Autodesk Inventor part; units mm, degrees
(part 7 of 8)
  spline S187 degree 3 poles (3.4162, -6.9877) (3.4167, -6.9758) (3.4179, -6.9524) (3.4233, -6.9183) (3.431, -6.8857) (3.4418, -6.8549) (3.4554, -6.8256) (3.4716, -6.7979) (3.4908, -6.7719) (3.5125, -6.7478) (3.5362, -6.7258) (3.5617, -6.7067) (3.5885, -6.6906) (3.6165, -6.6772) (3.6461, -6.6671) (3.6769, -6.6596) (3.7092, -6.6551) (3.7311, -6.6546) (3.7423, -6.6544) knots 0 0 0 0 0.068791 0.135103 0.198979 0.261904 0.323495 0.385195 0.446969 0.509765 0.572251 0.633405 0.693251 0.752583 0.812579 0.873275 0.93555 1 1 1 1
  spline S188 degree 3 poles (3.7423, -6.6544) (3.7532, -6.6546) (3.7748, -6.6551) (3.8062, -6.6595) (3.8362, -6.6662) (3.8645, -6.6758) (3.8911, -6.6886) (3.9161, -6.7039) (3.9398, -6.7217) (3.9611, -6.7426) (3.9807, -6.765) (3.9975, -6.7888) (4.012, -6.8135) (4.0241, -6.8391) (4.0329, -6.8659) (4.0397, -6.8935) (4.0435, -6.9223) (4.0441, -6.9417) (4.0444, -6.9516) knots 0 0 0 0 0.069475 0.136517 0.200789 0.26383 0.325735 0.387291 0.449509 0.512968 0.576275 0.63758 0.697903 0.757172 0.816599 0.876653 0.93729 1 1 1 1
  spline S189 degree 3 poles (4.0444, -6.9516) (4.0439, -6.9656) (4.0429, -6.9932) (4.0347, -7.0337) (4.0219, -7.0731) (4.0065, -7.1047) (3.9909, -7.1302) (3.9769, -7.1512) (3.9605, -7.1738) (3.9414, -7.1979) (3.9201, -7.2238) (3.8964, -7.2514) (3.8701, -7.2803) (3.8516, -7.3001) (3.842, -7.3104) knots 0 0 0 0 0.098702 0.195672 0.292422 0.391343 0.444462 0.504229 0.570352 0.642546 0.722288 0.807921 0.90047 1 1 1 1
  line L208 (3.842, -7.3104) -> (3.5918, -7.5774)
  line L209 (3.5918, -7.5774) -> (4.0572, -7.5774)
  line L210 (4.0572, -7.5774) -> (4.0572, -7.68)
  line L211 (4.0572, -7.68) -> (3.3777, -7.68)
  line L212 (3.3777, -7.68) -> (3.7655, -7.2661)
  spline S190 degree 3 poles (3.7655, -7.2661) (3.775, -7.2563) (3.7931, -7.2373) (3.8187, -7.2097) (3.8418, -7.1841) (3.8624, -7.1605) (3.88, -7.1386) (3.8957, -7.1191) (3.9083, -7.1012) (3.9219, -7.0804) (3.9351, -7.055) (3.9464, -7.024) (3.9534, -6.9921) (3.9542, -6.9705) (3.9546, -6.9596) knots 0 0 0 0 0.110803 0.212829 0.306101 0.390647 0.466924 0.534481 0.593587 0.644557 0.7362 0.825024 0.911986 1 1 1 1
  spline S191 degree 3 poles (3.1854, -6.9596) (3.1852, -6.9528) (3.1848, -6.9394) (3.1817, -6.9197) (3.1769, -6.9006) (3.1701, -6.8823) (3.161, -6.8647) (3.15, -6.848) (3.1374, -6.8318) (3.1227, -6.8166) (3.1066, -6.8027) (3.0895, -6.7903) (3.0715, -6.78) (3.0526, -6.7716) (3.0328, -6.765) (3.0121, -6.7604) (2.9906, -6.7575) (2.9759, -6.7571) (2.9684, -6.7569) knots 0 0 0 0 0.061965 0.122122 0.180988 0.239933 0.299906 0.359989 0.421776 0.486576 0.551535 0.615018 0.677259 0.73973 0.80305 0.866495 0.931973 1 1 1 1
  spline S192 degree 3 poles (2.9684, -6.7569) (2.9606, -6.7571) (2.9453, -6.7575) (2.9227, -6.7603) (2.9012, -6.7652) (2.8807, -6.7718) (2.8611, -6.7802) (2.8426, -6.7907) (2.8251, -6.8032) (2.8087, -6.8174) (2.7936, -6.8332) (2.7804, -6.8508) (2.7688, -6.8699) (2.7586, -6.8904) (2.7504, -6.9126) (2.7441, -6.9363) (2.7392, -6.9614) (2.7375, -6.9788) (2.7367, -6.9877) knots 0 0 0 0 0.064439 0.126547 0.186887 0.245878 0.304041 0.362191 0.420976 0.48066 0.5406 0.600689 0.661936 0.724443 0.789038 0.856314 0.926352 1 1 1 1
  line L213 (2.7367, -6.9877) -> (2.6469, -6.9877)
  spline S193 degree 3 poles (2.6469, -6.9877) (2.6475, -6.9758) (2.6487, -6.9524) (2.654, -6.9183) (2.6617, -6.8857) (2.6726, -6.8549) (2.6861, -6.8256) (2.7023, -6.7979) (2.7215, -6.7719) (2.7433, -6.7478) (2.767, -6.7258) (2.7925, -6.7067) (2.8193, -6.6906) (2.8473, -6.6772) (2.8769, -6.6671) (2.9077, -6.6596) (2.9399, -6.6551) (2.9619, -6.6546) (2.973, -6.6544) knots 0 0 0 0 0.068791 0.135103 0.198979 0.261904 0.323495 0.385195 0.446969 0.509765 0.572251 0.633405 0.693251 0.752583 0.812579 0.873275 0.93555 1 1 1 1
  spline S194 degree 3 poles (2.973, -6.6544) (2.984, -6.6546) (3.0056, -6.6551) (3.037, -6.6595) (3.0669, -6.6662) (3.0953, -6.6758) (3.1219, -6.6886) (3.1469, -6.7039) (3.1705, -6.7217) (3.1919, -6.7426) (3.2114, -6.765) (3.2283, -6.7888) (3.2428, -6.8135) (3.2548, -6.8391) (3.2637, -6.8659) (3.2704, -6.8935) (3.2742, -6.9223) (3.2748, -6.9417) (3.2751, -6.9516) knots 0 0 0 0 0.069475 0.136517 0.200789 0.26383 0.325735 0.387291 0.449509 0.512968 0.576275 0.63758 0.697903 0.757172 0.816599 0.876653 0.93729 1 1 1 1
  spline S195 degree 3 poles (3.2751, -6.9516) (3.2746, -6.9656) (3.2737, -6.9932) (3.2655, -7.0337) (3.2527, -7.0731) (3.2372, -7.1047) (3.2217, -7.1302) (3.2077, -7.1512) (3.1912, -7.1738) (3.1722, -7.1979) (3.1509, -7.2238) (3.1272, -7.2514) (3.1009, -7.2803) (3.0824, -7.3001) (3.0728, -7.3104) knots 0 0 0 0 0.098702 0.195672 0.292422 0.391343 0.444462 0.504229 0.570352 0.642546 0.722288 0.807921 0.90047 1 1 1 1
  line L214 (3.0728, -7.3104) -> (2.8226, -7.5774)
  line L215 (2.8226, -7.5774) -> (3.2879, -7.5774)
  line L216 (3.2879, -7.5774) -> (3.2879, -7.68)
  line L217 (3.2879, -7.68) -> (2.6085, -7.68)
  line L218 (2.6085, -7.68) -> (2.9963, -7.2661)
  spline S196 degree 3 poles (2.9963, -7.2661) (3.0057, -7.2563) (3.0239, -7.2373) (3.0495, -7.2097) (3.0726, -7.1841) (3.0931, -7.1605) (3.1108, -7.1386) (3.1265, -7.1191) (3.139, -7.1012) (3.1527, -7.0804) (3.1659, -7.055) (3.1772, -7.024) (3.1841, -6.9921) (3.185, -6.9705) (3.1854, -6.9596) knots 0 0 0 0 0.110803 0.212829 0.306101 0.390647 0.466924 0.534481 0.593587 0.644557 0.7362 0.825024 0.911986 1 1 1 1
  spline S197 degree 3 poles (7.9546, -4.4196) (7.9544, -4.4128) (7.9541, -4.3994) (7.9509, -4.3797) (7.9461, -4.3606) (7.9393, -4.3423) (7.9303, -4.3247) (7.9193, -4.308) (7.9066, -4.2918) (7.8919, -4.2766) (7.8758, -4.2627) (7.8588, -4.2503) (7.8408, -4.24) (7.8218, -4.2316) (7.8021, -4.225) (7.7814, -4.2204) (7.7599, -4.2175) (7.7452, -4.2171) (7.7377, -4.2169) knots 0 0 0 0 0.061965 0.122122 0.180988 0.239933 0.299906 0.359989 0.421776 0.486576 0.551535 0.615018 0.677259 0.73973 0.80305 0.866495 0.931973 1 1 1 1
  spline S198 degree 3 poles (7.7377, -4.2169) (7.7298, -4.2171) (7.7145, -4.2175) (7.6919, -4.2203) (7.6704, -4.2252) (7.6499, -4.2318) (7.6303, -4.2402) (7.6118, -4.2507) (7.5943, -4.2632) (7.578, -4.2774) (7.5629, -4.2932) (7.5496, -4.3108) (7.538, -4.3299) (7.5279, -4.3504) (7.5197, -4.3726) (7.5134, -4.3963) (7.5084, -4.4214) (7.5067, -4.4388) (7.5059, -4.4477) knots 0 0 0 0 0.064439 0.126547 0.186887 0.245878 0.304041 0.362191 0.420976 0.48066 0.5406 0.600689 0.661936 0.724443 0.789038 0.856314 0.926352 1 1 1 1
  line L219 (7.5059, -4.4477) -> (7.4162, -4.4477)
  spline S199 degree 3 poles (7.4162, -4.4477) (7.4167, -4.4358) (7.4179, -4.4124) (7.4233, -4.3783) (7.431, -4.3457) (7.4418, -4.3149) (7.4554, -4.2856) (7.4716, -4.2579) (7.4908, -4.2319) (7.5125, -4.2078) (7.5362, -4.1858) (7.5617, -4.1667) (7.5885, -4.1506) (7.6165, -4.1372) (7.6461, -4.1271) (7.6769, -4.1196) (7.7092, -4.1151) (7.7311, -4.1146) (7.7423, -4.1144) knots 0 0 0 0 0.068791 0.135103 0.198979 0.261904 0.323495 0.385195 0.446969 0.509765 0.572251 0.633405 0.693251 0.752583 0.812579 0.873275 0.93555 1 1 1 1
  spline S200 degree 3 poles (7.7423, -4.1144) (7.7532, -4.1146) (7.7748, -4.1151) (7.8062, -4.1195) (7.8362, -4.1262) (7.8645, -4.1358) (7.8911, -4.1486) (7.9161, -4.1639) (7.9398, -4.1817) (7.9611, -4.2026) (7.9807, -4.225) (7.9975, -4.2488) (8.012, -4.2735) (8.0241, -4.2991) (8.0329, -4.3259) (8.0397, -4.3535) (8.0435, -4.3823) (8.0441, -4.4017) (8.0444, -4.4116) knots 0 0 0 0 0.069475 0.136517 0.200789 0.26383 0.325735 0.387291 0.449509 0.512968 0.576275 0.63758 0.697903 0.757172 0.816599 0.876653 0.93729 1 1 1 1
  spline S201 degree 3 poles (8.0444, -4.4116) (8.0439, -4.4256) (8.0429, -4.4532) (8.0347, -4.4937) (8.0219, -4.5331) (8.0065, -4.5647) (7.9909, -4.5902) (7.9769, -4.6112) (7.9605, -4.6338) (7.9414, -4.6579) (7.9201, -4.6838) (7.8964, -4.7114) (7.8701, -4.7403) (7.8516, -4.7601) (7.842, -4.7704) knots 0 0 0 0 0.098702 0.195672 0.292422 0.391343 0.444462 0.504229 0.570352 0.642546 0.722288 0.807921 0.90047 1 1 1 1
  line L220 (7.842, -4.7704) -> (7.5918, -5.0374)
  line L221 (7.5918, -5.0374) -> (8.0572, -5.0374)
  line L222 (8.0572, -5.0374) -> (8.0572, -5.14)
  line L223 (8.0572, -5.14) -> (7.3777, -5.14)
  line L224 (7.3777, -5.14) -> (7.7655, -4.7261)
  spline S202 degree 3 poles (7.7655, -4.7261) (7.775, -4.7163) (7.7931, -4.6973) (7.8187, -4.6697) (7.8418, -4.6441) (7.8624, -4.6205) (7.88, -4.5986) (7.8957, -4.5791) (7.9083, -4.5612) (7.9219, -4.5404) (7.9351, -4.515) (7.9464, -4.484) (7.9534, -4.4521) (7.9542, -4.4305) (7.9546, -4.4196) knots 0 0 0 0 0.110803 0.212829 0.306101 0.390647 0.466924 0.534481 0.593587 0.644557 0.7362 0.825024 0.911986 1 1 1 1
  spline S203 degree 3 poles (7.1469, -4.3738) (7.1468, -4.3686) (7.1466, -4.3582) (7.1436, -4.343) (7.1391, -4.3283) (7.133, -4.3141) (7.1248, -4.3005) (7.115, -4.2875) (7.1032, -4.275) (7.0898, -4.2634) (7.0754, -4.2523) (7.0596, -4.2429) (7.043, -4.2349) (7.0253, -4.2282) (7.0067, -4.2232) (6.9872, -4.2196) (6.9668, -4.2174) (6.9529, -4.2171) (6.9458, -4.2169) knots 0 0 0 0 0.055275 0.109966 0.163247 0.218076 0.273301 0.330909 0.390995 0.454176 0.518862 0.583311 0.648517 0.715031 0.782502 0.852323 0.924928 1 1 1 1
  spline S204 degree 3 poles (6.9458, -4.2169) (6.9344, -4.2173) (6.9122, -4.2181) (6.8801, -4.2249) (6.8503, -4.2357) (6.8275, -4.2487) (6.8107, -4.2615) (6.7987, -4.2727) (6.7869, -4.2851) (6.7761, -4.2995) (6.7651, -4.3149) (6.7552, -4.3322) (6.7455, -4.3508) (6.7397, -4.364) (6.7367, -4.3708) knots 0 0 0 0 0.122712 0.239685 0.351816 0.463766 0.520818 0.579448 0.640604 0.705298 0.773634 0.844669 0.920057 1 1 1 1
  line L225 (6.7367, -4.3708) -> (6.6469, -4.3708)
  spline S205 degree 3 poles (6.6469, -4.3708) (6.6494, -4.3607) (6.6541, -4.341) (6.664, -4.3129) (6.6748, -4.2863) (6.6878, -4.2617) (6.7019, -4.2386) (6.7181, -4.2176) (6.7357, -4.198) (6.755, -4.1807) (6.7754, -4.165) (6.7969, -4.1516) (6.8193, -4.1401) (6.8426, -4.1306) (6.8669, -4.1234) (6.892, -4.1182) (6.918, -4.1149) (6.9356, -4.1145) (6.9446, -4.1144) knots 0 0 0 0 0.072625 0.141977 0.208985 0.273957 0.336889 0.398745 0.460116 0.520825 0.580994 0.640152 0.698622 0.757271 0.816427 0.876254 0.937165 1 1 1 1
  spline S206 degree 3 poles (6.9446, -4.1144) (6.9577, -4.1148) (6.9835, -4.1155) (7.0214, -4.1227) (7.058, -4.1339) (7.0928, -4.1495) (7.1252, -4.1687) (7.1539, -4.1915) (7.1788, -4.2176) (7.1996, -4.2464) (7.2159, -4.2771) (7.2279, -4.3088) (7.2352, -4.3413) (7.2362, -4.3632) (7.2367, -4.3742) knots 0 0 0 0 0.090254 0.17854 0.266093 0.354631 0.441886 0.525747 0.608114 0.690197 0.770821 0.848326 0.924012 1 1 1 1
  spline S207 degree 3 poles (7.2367, -4.3742) (7.2363, -4.3847) (7.2357, -4.4054) (7.2302, -4.4356) (7.2209, -4.4641) (7.208, -4.491) (7.1913, -4.516) (7.1711, -4.5394) (7.1473, -4.5611) (7.1292, -4.5735) (7.1199, -4.5799) knots 0 0 0 0 0.128068 0.250608 0.37063 0.490072 0.610375 0.734313 0.863217 1 1 1 1
  spline S208 degree 3 poles (7.1199, -4.5799) (7.1305, -4.585) (7.1516, -4.5952) (7.1803, -4.6152) (7.2064, -4.6382) (7.2209, -4.6562) (7.2283, -4.6652) knots 0 0 0 0 0.25388 0.503009 0.750291 1 1 1 1
  spline S209 degree 3 poles (7.2283, -4.6652) (7.2331, -4.6718) (7.2426, -4.6849) (7.2544, -4.7059) (7.2651, -4.7271) (7.2734, -4.7492) (7.2799, -4.7718) (7.2845, -4.795) (7.2873, -4.8187) (7.2877, -4.8348) (7.2879, -4.8429) knots 0 0 0 0 0.128136 0.254173 0.378112 0.501712 0.623986 0.747096 0.872875 1 1 1 1
  spline S210 degree 3 poles (7.2879, -4.8429) (7.2874, -4.8569) (7.2864, -4.8849) (7.2773, -4.9261) (7.2631, -4.9665) (7.243, -5.0051) (7.2184, -5.0412) (7.1892, -5.0735) (7.1557, -5.1013) (7.1184, -5.1245) (7.0779, -5.143) (7.0346, -5.1559) (6.9891, -5.1643) (6.9579, -5.1652) (6.942, -5.1656) knots 0 0 0 0 0.079648 0.158922 0.239619 0.322609 0.406035 0.487602 0.569685 0.653036 0.737436 0.822478 0.909748 1 1 1 1
  spline S211 degree 3 poles (6.942, -5.1656) (6.9313, -5.1654) (6.9103, -5.1649) (6.8793, -5.1616) (6.8498, -5.1555) (6.8217, -5.1473) (6.7949, -5.1369) (6.7695, -5.1239) (6.7453, -5.1087) (6.7227, -5.091) (6.7016, -5.0712) (6.6825, -5.049) (6.6652, -5.0247) (6.6501, -4.9981) (6.6364, -4.9695) (6.6252, -4.9386) (6.6154, -4.9056) (6.6108, -4.8826) (6.6085, -4.8708) knots 0 0 0 0 0.065541 0.128963 0.190377 0.250092 0.308548 0.366398 0.424542 0.48317 0.542243 0.601739 0.662506 0.724856 0.789128 0.856346 0.926295 1 1 1 1
  line L226 (6.6085, -4.8708) -> (6.6982, -4.8708)
  spline S212 degree 3 poles (6.6982, -4.8708) (6.7005, -4.8785) (6.7051, -4.8934) (6.7128, -4.915) (6.7217, -4.9348) (6.7311, -4.9529) (6.741, -4.9695) (6.7522, -4.9842) (6.7636, -4.9977) (6.7723, -5.0053) (6.7765, -5.009) knots 0 0 0 0 0.14977 0.291316 0.425966 0.55216 0.671527 0.786122 0.895325 1 1 1 1
  spline S213 degree 3 poles (6.7765, -5.009) (6.7821, -5.0133) (6.7933, -5.0219) (6.8115, -5.0329) (6.8307, -5.0425) (6.8512, -5.0497) (6.8726, -5.0559) (6.8953, -5.0599) (6.9191, -5.0627) (6.9353, -5.063) (6.9436, -5.0631) knots 0 0 0 0 0.118271 0.236178 0.355663 0.475904 0.600127 0.728608 0.861313 1 1 1 1
  spline S214 degree 3 poles (6.9436, -5.0631) (6.953, -5.0629) (6.9713, -5.0626) (6.998, -5.0594) (7.0234, -5.0548) (7.0472, -5.0477) (7.0697, -5.0389) (7.0907, -5.0278) (7.1104, -5.0149) (7.1284, -5.0001) (7.1447, -4.984) (7.159, -4.9672) (7.1712, -4.9496) (7.181, -4.9313) (7.1888, -4.9124) (7.1941, -4.8926) (7.1978, -4.8723) (7.1981, -4.8585) (7.1982, -4.8515) knots 0 0 0 0 0.076072 0.148752 0.218403 0.28576 0.350598 0.414964 0.478069 0.541761 0.60435 0.664075 0.721464 0.777587 0.832644 0.887844 0.94346 1 1 1 1
  spline S215 degree 3 poles (7.1982, -4.8515) (7.1978, -4.8422) (7.1969, -4.8236) (7.1902, -4.7963) (7.1793, -4.7699) (7.1639, -4.745) (7.1453, -4.722) (7.1235, -4.7014) (7.0983, -4.6844) (7.0752, -4.6726) (7.0547, -4.6646) (7.0371, -4.6593) (7.0175, -4.6548) (6.996, -4.6506) (6.9724, -4.647) (6.9469, -4.644) (6.9194, -4.6416) (6.9003, -4.6405) (6.8905, -4.64) knots 0 0 0 0 0.066909 0.133485 0.201035 0.271234 0.34288 0.413836 0.485977 0.56023 0.599884 0.644055 0.691892 0.744688 0.801492 0.862858 0.929328 1 1 1 1
  line L227 (6.8905, -4.64) -> (6.8905, -4.5374)
  spline S216 degree 3 poles (6.8905, -4.5374) (6.9029, -4.5372) (6.9271, -4.5368) (6.9625, -4.5318) (6.9964, -4.525) (7.0279, -4.5144) (7.0567, -4.5022) (7.0816, -4.4879) (7.1024, -4.4721) (7.1189, -4.4544) (7.1314, -4.4355) (7.1405, -4.4157) (7.1458, -4.395) (7.1466, -4.3809) (7.1469, -4.3738) knots 0 0 0 0 0.110166 0.215787 0.318027 0.417574 0.51165 0.596162 0.672935 0.74367 0.810677 0.874059 0.936696 1 1 1 1
  line L228 (3.6854, -4.2426) -> (3.5315, -4.2426)
  line L229 (3.5315, -4.2426) -> (3.5902, -4.14)
  line L230 (3.5902, -4.14) -> (3.7751, -4.14)
  line L231 (3.7751, -4.14) -> (3.7751, -5.14)
  line L232 (3.7751, -5.14) -> (3.6854, -5.14)
  line L233 (3.6854, -5.14) -> (3.6854, -4.2426)
  spline S217 degree 3 poles (3.1854, -4.4196) (3.1852, -4.4128) (3.1848, -4.3994) (3.1817, -4.3797) (3.1769, -4.3606) (3.1701, -4.3423) (3.161, -4.3247) (3.15, -4.308) (3.1374, -4.2918) (3.1227, -4.2766) (3.1066, -4.2627) (3.0895, -4.2503) (3.0715, -4.24) (3.0526, -4.2316) (3.0328, -4.225) (3.0121, -4.2204) (2.9906, -4.2175) (2.9759, -4.2171) (2.9684, -4.2169) knots 0 0 0 0 0.061965 0.122122 0.180988 0.239933 0.299906 0.359989 0.421776 0.486576 0.551535 0.615018 0.677259 0.73973 0.80305 0.866495 0.931973 1 1 1 1
  spline S218 degree 3 poles (2.9684, -4.2169) (2.9606, -4.2171) (2.9453, -4.2175) (2.9227, -4.2203) (2.9012, -4.2252) (2.8807, -4.2318) (2.8611, -4.2402) (2.8426, -4.2507) (2.8251, -4.2632) (2.8087, -4.2774) (2.7936, -4.2932) (2.7804, -4.3108) (2.7688, -4.3299) (2.7586, -4.3504) (2.7504, -4.3726) (2.7441, -4.3963) (2.7392, -4.4214) (2.7375, -4.4388) (2.7367, -4.4477) knots 0 0 0 0 0.064439 0.126547 0.186887 0.245878 0.304041 0.362191 0.420976 0.48066 0.5406 0.600689 0.661936 0.724443 0.789038 0.856314 0.926352 1 1 1 1
  line L234 (2.7367, -4.4477) -> (2.6469, -4.4477)
  spline S219 degree 3 poles (2.6469, -4.4477) (2.6475, -4.4358) (2.6487, -4.4124) (2.654, -4.3783) (2.6617, -4.3457) (2.6726, -4.3149) (2.6861, -4.2856) (2.7023, -4.2579) (2.7215, -4.2319) (2.7433, -4.2078) (2.767, -4.1858) (2.7925, -4.1667) (2.8193, -4.1506) (2.8473, -4.1372) (2.8769, -4.1271) (2.9077, -4.1196) (2.9399, -4.1151) (2.9619, -4.1146) (2.973, -4.1144) knots 0 0 0 0 0.068791 0.135103 0.198979 0.261904 0.323495 0.385195 0.446969 0.509765 0.572251 0.633405 0.693251 0.752583 0.812579 0.873275 0.93555 1 1 1 1
  spline S220 degree 3 poles (2.973, -4.1144) (2.984, -4.1146) (3.0056, -4.1151) (3.037, -4.1195) (3.0669, -4.1262) (3.0953, -4.1358) (3.1219, -4.1486) (3.1469, -4.1639) (3.1705, -4.1817) (3.1919, -4.2026) (3.2114, -4.225) (3.2283, -4.2488) (3.2428, -4.2735) (3.2548, -4.2991) (3.2637, -4.3259) (3.2704, -4.3535) (3.2742, -4.3823) (3.2748, -4.4017) (3.2751, -4.4116) knots 0 0 0 0 0.069475 0.136517 0.200789 0.26383 0.325735 0.387291 0.449509 0.512968 0.576275 0.63758 0.697903 0.757172 0.816599 0.876653 0.93729 1 1 1 1
  spline S221 degree 3 poles (3.2751, -4.4116) (3.2746, -4.4256) (3.2737, -4.4532) (3.2655, -4.4937) (3.2527, -4.5331) (3.2372, -4.5647) (3.2217, -4.5902) (3.2077, -4.6112) (3.1912, -4.6338) (3.1722, -4.6579) (3.1509, -4.6838) (3.1272, -4.7114) (3.1009, -4.7403) (3.0824, -4.7601) (3.0728, -4.7704) knots 0 0 0 0 0.098702 0.195672 0.292422 0.391343 0.444462 0.504229 0.570352 0.642546 0.722288 0.807921 0.90047 1 1 1 1
  line L235 (3.0728, -4.7704) -> (2.8226, -5.0374)
  line L236 (2.8226, -5.0374) -> (3.2879, -5.0374)
  line L237 (3.2879, -5.0374) -> (3.2879, -5.14)
  line L238 (3.2879, -5.14) -> (2.6085, -5.14)
  line L239 (2.6085, -5.14) -> (2.9963, -4.7261)
  spline S222 degree 3 poles (2.9963, -4.7261) (3.0057, -4.7163) (3.0239, -4.6973) (3.0495, -4.6697) (3.0726, -4.6441) (3.0931, -4.6205) (3.1108, -4.5986) (3.1265, -4.5791) (3.139, -4.5612) (3.1527, -4.5404) (3.1659, -4.515) (3.1772, -4.484) (3.1841, -4.4521) (3.185, -4.4305) (3.1854, -4.4196) knots 0 0 0 0 0.110803 0.212829 0.306101 0.390647 0.466924 0.534481 0.593587 0.644557 0.7362 0.825024 0.911986 1 1 1 1
  spline S223 degree 3 poles (7.9546, -1.8796) (7.9544, -1.8728) (7.9541, -1.8594) (7.9509, -1.8397) (7.9461, -1.8206) (7.9393, -1.8023) (7.9303, -1.7847) (7.9193, -1.768) (7.9066, -1.7518) (7.8919, -1.7366) (7.8758, -1.7227) (7.8588, -1.7103) (7.8408, -1.7) (7.8218, -1.6916) (7.8021, -1.685) (7.7814, -1.6804) (7.7599, -1.6775) (7.7452, -1.6771) (7.7377, -1.6769) knots 0 0 0 0 0.061965 0.122122 0.180988 0.239933 0.299906 0.359989 0.421776 0.486576 0.551535 0.615018 0.677259 0.73973 0.80305 0.866495 0.931973 1 1 1 1
  spline S224 degree 3 poles (7.7377, -1.6769) (7.7298, -1.6771) (7.7145, -1.6775) (7.6919, -1.6803) (7.6704, -1.6852) (7.6499, -1.6918) (7.6303, -1.7002) (7.6118, -1.7107) (7.5943, -1.7232) (7.578, -1.7374) (7.5629, -1.7532) (7.5496, -1.7708) (7.538, -1.7899) (7.5279, -1.8104) (7.5197, -1.8326) (7.5134, -1.8563) (7.5084, -1.8814) (7.5067, -1.8988) (7.5059, -1.9077) knots 0 0 0 0 0.064439 0.126547 0.186887 0.245878 0.304041 0.362191 0.420976 0.48066 0.5406 0.600689 0.661936 0.724443 0.789038 0.856314 0.926352 1 1 1 1
  line L240 (7.5059, -1.9077) -> (7.4162, -1.9077)
  spline S225 degree 3 poles (7.4162, -1.9077) (7.4167, -1.8958) (7.4179, -1.8724) (7.4233, -1.8383) (7.431, -1.8057) (7.4418, -1.7749) (7.4554, -1.7456) (7.4716, -1.7179) (7.4908, -1.6919) (7.5125, -1.6678) (7.5362, -1.6458) (7.5617, -1.6267) (7.5885, -1.6106) (7.6165, -1.5972) (7.6461, -1.5871) (7.6769, -1.5796) (7.7092, -1.5751) (7.7311, -1.5746) (7.7423, -1.5744) knots 0 0 0 0 0.068791 0.135103 0.198979 0.261904 0.323495 0.385195 0.446969 0.509765 0.572251 0.633405 0.693251 0.752583 0.812579 0.873275 0.93555 1 1 1 1
  spline S226 degree 3 poles (7.7423, -1.5744) (7.7532, -1.5746) (7.7748, -1.5751) (7.8062, -1.5795) (7.8362, -1.5862) (7.8645, -1.5958) (7.8911, -1.6086) (7.9161, -1.6239) (7.9398, -1.6417) (7.9611, -1.6626) (7.9807, -1.685) (7.9975, -1.7088) (8.012, -1.7335) (8.0241, -1.7591) (8.0329, -1.7859) (8.0397, -1.8135) (8.0435, -1.8423) (8.0441, -1.8617) (8.0444, -1.8716) knots 0 0 0 0 0.069475 0.136517 0.200789 0.26383 0.325735 0.387291 0.449509 0.512968 0.576275 0.63758 0.697903 0.757172 0.816599 0.876653 0.93729 1 1 1 1
  spline S227 degree 3 poles (8.0444, -1.8716) (8.0439, -1.8856) (8.0429, -1.9132) (8.0347, -1.9537) (8.0219, -1.9931) (8.0065, -2.0247) (7.9909, -2.0502) (7.9769, -2.0712) (7.9605, -2.0938) (7.9414, -2.1179) (7.9201, -2.1438) (7.8964, -2.1714) (7.8701, -2.2003) (7.8516, -2.2201) (7.842, -2.2304) knots 0 0 0 0 0.098702 0.195672 0.292422 0.391343 0.444462 0.504229 0.570352 0.642546 0.722288 0.807921 0.90047 1 1 1 1
  line L241 (7.842, -2.2304) -> (7.5918, -2.4974)
  line L242 (7.5918, -2.4974) -> (8.0572, -2.4974)
  line L243 (8.0572, -2.4974) -> (8.0572, -2.6)
  line L244 (8.0572, -2.6) -> (7.3777, -2.6)
  line L245 (7.3777, -2.6) -> (7.7655, -2.1861)
  spline S228 degree 3 poles (7.7655, -2.1861) (7.775, -2.1763) (7.7931, -2.1573) (7.8187, -2.1297) (7.8418, -2.1041) (7.8624, -2.0805) (7.88, -2.0586) (7.8957, -2.0391) (7.9083, -2.0212) (7.9219, -2.0004) (7.9351, -1.975) (7.9464, -1.944) (7.9534, -1.9121) (7.9542, -1.8905) (7.9546, -1.8796) knots 0 0 0 0 0.110803 0.212829 0.306101 0.390647 0.466924 0.534481 0.593587 0.644557 0.7362 0.825024 0.911986 1 1 1 1
  line L246 (6.9162, -1.7026) -> (6.7623, -1.7026)
  line L247 (6.7623, -1.7026) -> (6.821, -1.6)
  line L248 (6.821, -1.6) -> (7.0059, -1.6)
  line L249 (7.0059, -1.6) -> (7.0059, -2.6)
  line L250 (7.0059, -2.6) -> (6.9162, -2.6)
  line L251 (6.9162, -2.6) -> (6.9162, -1.7026)
  line L252 (3.9053, -1.7026) -> (3.4418, -1.7026)
  line L253 (3.4418, -1.7026) -> (3.4418, -1.6)
  line L254 (3.4418, -1.6) -> (4.0572, -1.6)
  line L255 (4.0572, -1.6) -> (3.5315, -2.6256)
  line L256 (3.5315, -2.6256) -> (3.454, -2.583)
  line L257 (3.454, -2.583) -> (3.9053, -1.7026)
  line L258 (2.9162, -1.7026) -> (2.7623, -1.7026)
  line L259 (2.7623, -1.7026) -> (2.821, -1.6)
  line L260 (2.821, -1.6) -> (3.0059, -1.6)
  line L261 (3.0059, -1.6) -> (3.0059, -2.6)
  line L262 (3.0059, -2.6) -> (2.9162, -2.6)
  line L263 (2.9162, -2.6) -> (2.9162, -1.7026)
  line L264 (7.8521, 0.1708) -> (7.3777, 0.1708)
  line L265 (7.3777, 0.1708) -> (7.9236, 0.9656)
  line L266 (7.9236, 0.9656) -> (7.9418, 0.9656)
  line L267 (7.9418, 0.9656) -> (7.9418, 0.2733)
  line L268 (7.9418, 0.2733) -> (8.0572, 0.2733)
  line L269 (8.0572, 0.2733) -> (8.0572, 0.1708)
  line L270 (8.0572, 0.1708) -> (7.9418, 0.1708)
  line L271 (7.9418, 0.1708) -> (7.9418, -0.06)
  line L272 (7.9418, -0.06) -> (7.8521, -0.06)
  line L273 (7.8521, -0.06) -> (7.8521, 0.1708)
  spline S229 degree 3 poles (3.429, 0.2188) (3.4293, 0.2291) (3.43, 0.2502) (3.4348, 0.282) (3.4425, 0.3146) (3.4512, 0.3422) (3.4604, 0.3649) (3.468, 0.3832) (3.4774, 0.4019) (3.4876, 0.4219) (3.4992, 0.4425) (3.5119, 0.4642) (3.5259, 0.4865) (3.5357, 0.5016) (3.5408, 0.5093) knots 0 0 0 0 0.097818 0.199726 0.305276 0.415811 0.474472 0.537274 0.603657 0.674299 0.749834 0.828598 0.912378 1 1 1 1
  line L274 (3.5408, 0.5093) -> (3.8392, 0.9656)
  line L275 (3.8392, 0.9656) -> (3.9083, 0.9114)
  line L276 (3.9083, 0.9114) -> (3.6441, 0.5073)
  spline S230 degree 3 poles (3.6441, 0.5073) (3.6617, 0.5101) (3.696, 0.5156) (3.7308, 0.5165) (3.7477, 0.5169) knots 0 0 0 0 0.512659 1 1 1 1
  spline S231 degree 3 poles (3.7477, 0.5169) (3.7578, 0.5166) (3.7779, 0.5161) (3.8072, 0.512) (3.8355, 0.5055) (3.8624, 0.4959) (3.8882, 0.4838) (3.913, 0.4692) (3.9363, 0.4515) (3.9584, 0.4317) (3.9784, 0.4098) (3.9962, 0.3866) (4.0111, 0.362) (4.0232, 0.3361) (4.0326, 0.309) (4.0395, 0.2806) (4.0435, 0.251) (4.0441, 0.2309) (4.0444, 0.2206) knots 0 0 0 0 0.065231 0.128405 0.190067 0.250943 0.311546 0.372863 0.435024 0.499072 0.563091 0.62551 0.68668 0.747283 0.808563 0.870742 0.934341 1 1 1 1
  spline S232 degree 3 poles (4.0444, 0.2206) (4.044, 0.2067) (4.0432, 0.1791) (4.0352, 0.139) (4.0228, 0.1008) (4.0051, 0.0651) (3.9831, 0.032) (3.9563, 0.0026) (3.9256, -0.0236) (3.8909, -0.0455) (3.8535, -0.0634) (3.8143, -0.0762) (3.7735, -0.0841) (3.7459, -0.0851) (3.7319, -0.0856) knots 0 0 0 0 0.085948 0.169125 0.250399 0.33229 0.413364 0.494172 0.576022 0.660757 0.745783 0.830044 0.914028 1 1 1 1
  spline S233 degree 3 poles (3.7319, -0.0856) (3.7184, -0.0852) (3.6917, -0.0843) (3.6525, -0.0766) (3.6149, -0.0641) (3.579, -0.0469) (3.5458, -0.0252) (3.516, 0.0009) (3.4899, 0.031) (3.4682, 0.0649) (3.451, 0.1013) (3.4381, 0.1393) (3.4306, 0.1787) (3.4295, 0.2054) (3.429, 0.2188) knots 0 0 0 0 0.084335 0.167052 0.249566 0.33274 0.415915 0.497828 0.580373 0.6646 0.749467 0.83251 0.915639 1 1 1 1
  spline S234 degree 3 poles (7.2879, 2.9796) (7.2878, 2.9643) (7.2874, 2.9345) (7.2855, 2.8909) (7.2818, 2.8498) (7.2772, 2.811) (7.2708, 2.7747) (7.2629, 2.7408) (7.2541, 2.7091) (7.2433, 2.6798) (7.2315, 2.6527) (7.2186, 2.6274) (7.2048, 2.6036) (7.1898, 2.5816) (7.1738, 2.5612) (7.1564, 2.5428) (7.1382, 2.5259) (7.119, 2.5109) (7.0989, 2.4977) (7.0783, 2.4859) (7.0569, 2.4764) (7.0352, 2.4683) (7.0129, 2.462) (6.99, 2.4577) (6.9666, 2.4547) (6.9508, 2.4545) (6.9428, 2.4544) knots 0 0 0 0 0.065063 0.126773 0.185516 0.240765 0.29298 0.34225 0.388919 0.432776 0.474628 0.514775 0.553606 0.591426 0.628028 0.663804 0.698984 0.733591 0.767628 0.801208 0.834264 0.866981 0.89972 0.932702 0.966176 1 1 1 1
  spline S235 degree 3 poles (6.9428, 2.4544) (6.9349, 2.4545) (6.9194, 2.4548) (6.8963, 2.4575) (6.8739, 2.4618) (6.8521, 2.468) (6.8308, 2.4755) (6.8102, 2.4852) (6.7901, 2.4964) (6.7706, 2.5092) (6.752, 2.5239) (6.7343, 2.5401) (6.7178, 2.5583) (6.7025, 2.5782) (6.6879, 2.5995) (6.6745, 2.6226) (6.6622, 2.6474) (6.6508, 2.6741) (6.6408, 2.703) (6.6319, 2.7345) (6.6249, 2.7688) (6.6189, 2.8057) (6.6141, 2.8453) (6.6108, 2.8877) (6.6087, 2.9328) (6.6086, 2.9637) (6.6085, 2.9796) knots 0 0 0 0 0.033787 0.066622 0.099285 0.131361 0.163585 0.196104 0.228902 0.262158 0.295991 0.330218 0.36506 0.400951 0.43762 0.475708 0.515381 0.556414 0.599765 0.646424 0.696431 0.749782 0.806573 0.867436 0.931887 1 1 1 1
  spline S236 degree 3 poles (6.6085, 2.9796) (6.6086, 2.9956) (6.6087, 3.0268) (6.6108, 3.0721) (6.6141, 3.1147) (6.6187, 3.1544) (6.6243, 3.1914) (6.6318, 3.2255) (6.6404, 3.2568) (6.6502, 3.2855) (6.6614, 3.312) (6.6735, 3.3366) (6.6871, 3.3595) (6.7014, 3.381) (6.7169, 3.4007) (6.7333, 3.4189) (6.7511, 3.4351) (6.7698, 3.45) (6.7895, 3.4629) (6.8097, 3.4744) (6.8305, 3.4841) (6.8519, 3.4918) (6.8739, 3.4982) (6.8963, 3.5025) (6.9194, 3.5052) (6.9349, 3.5055) (6.9428, 3.5056) knots 0 0 0 0 0.068595 0.133246 0.194313 0.251279 0.304513 0.354235 0.400481 0.443411 0.484015 0.523252 0.561042 0.5979 0.633518 0.668314 0.702496 0.736685 0.770293 0.803437 0.835913 0.86846 0.900847 0.933467 0.966258 1 1 1 1
  spline S237 degree 3 poles (6.9428, 3.5056) (6.9507, 3.5055) (6.9666, 3.5052) (6.9899, 3.5026) (7.0128, 3.4981) (7.035, 3.4919) (7.0567, 3.4841) (7.0779, 3.4744) (7.0985, 3.463) (7.1183, 3.4497) (7.1375, 3.4349) (7.1556, 3.4181) (7.1727, 3.3995) (7.1889, 3.3794) (7.2038, 3.3573) (7.2179, 3.3337) (7.2306, 3.308) (7.2428, 3.2808) (7.2534, 3.2513) (7.2629, 3.2197) (7.2705, 3.1855) (7.2769, 3.149) (7.2819, 3.11) (7.2855, 3.0687) (7.2874, 3.0249) (7.2878, 2.995) (7.2879, 2.9796) knots 0 0 0 0 0.033788 0.067194 0.099862 0.132567 0.165151 0.197913 0.231319 0.265083 0.299255 0.334399 0.369943 0.406284 0.444064 0.482998 0.523354 0.565537 0.609613 0.656391 0.705885 0.758325 0.813832 0.872795 0.934722 1 1 1 1
  line L277 (3.9931, 3.2653) -> (3.9931, 2.48)
  line L278 (3.9931, 2.48) -> (3.9033, 2.48)
  line L279 (3.9033, 2.48) -> (3.9033, 3.48)
  line L280 (3.9033, 3.48) -> (3.9222, 3.48)
  line L281 (3.9222, 3.48) -> (4.5828, 2.6929)
  line L282 (4.5828, 2.6929) -> (4.5828, 3.48)
  line L283 (4.5828, 3.48) -> (4.6726, 3.48)
  line L284 (4.6726, 3.48) -> (4.6726, 2.48)
  line L285 (4.6726, 2.48) -> (4.6521, 2.48)
  line L286 (4.6521, 2.48) -> (3.9931, 3.2653)
  spline S238 degree 3 poles (2.6469, 2.9804) (2.6471, 2.9922) (2.6474, 3.0155) (2.651, 3.0502) (2.6563, 3.0843) (2.664, 3.1178) (2.6738, 3.1506) (2.6859, 3.1828) (2.7001, 3.2144) (2.7165, 3.2452) (2.7348, 3.2749) (2.7547, 3.3031) (2.7764, 3.3296) (2.7996, 3.3545) (2.8246, 3.3776) (2.8511, 3.399) (2.8792, 3.4189) (2.9089, 3.4369) (2.9398, 3.4531) (2.9718, 3.4672) (3.0049, 3.4789) (3.0389, 3.4889) (3.074, 3.4962) (3.11, 3.5016) (3.147, 3.5052) (3.1721, 3.5055) (3.1848, 3.5056) knots 0 0 0 0 0.042039 0.083544 0.124643 0.165303 0.206171 0.246971 0.288329 0.329987 0.371797 0.412738 0.453459 0.494001 0.534381 0.574952 0.615892 0.65725 0.699007 0.740486 0.782325 0.824567 0.867041 0.9105 0.954619 1 1 1 1
  spline S239 degree 3 poles (3.1848, 3.5056) (3.1951, 3.5055) (3.2157, 3.5051) (3.2462, 3.5029) (3.2763, 3.4993) (3.3059, 3.4943) (3.3351, 3.4876) (3.3637, 3.4796) (3.392, 3.4703) (3.4198, 3.4591) (3.4473, 3.4465) (3.4746, 3.4323) (3.5017, 3.4162) (3.5285, 3.3983) (3.5554, 3.3787) (3.5818, 3.3571) (3.6083, 3.3342) (3.6254, 3.3177) (3.6341, 3.3093) knots 0 0 0 0 0.061617 0.122179 0.182216 0.241864 0.30096 0.359969 0.419033 0.478069 0.537993 0.59896 0.661321 0.725248 0.79122 0.858746 0.928318 1 1 1 1
  line L287 (3.6341, 3.3093) -> (3.5572, 3.2364)
  spline S240 degree 3 poles (3.5572, 3.2364) (3.5433, 3.2495) (3.5158, 3.2754) (3.4709, 3.309) (3.4241, 3.3377) (3.3756, 3.3611) (3.3266, 3.3798) (3.2778, 3.3931) (3.2296, 3.4016) (3.1976, 3.4026) (3.1818, 3.4031) knots 0 0 0 0 0.136144 0.269043 0.398517 0.5271 0.652283 0.77168 0.887495 1 1 1 1
  spline S241 degree 3 poles (3.1818, 3.4031) (3.1721, 3.403) (3.1527, 3.4027) (3.124, 3.3997) (3.0955, 3.3954) (3.0674, 3.3891) (3.0397, 3.3812) (3.0123, 3.3712) (2.9852, 3.3596) (2.9588, 3.3462) (2.9331, 3.3315) (2.9089, 3.3152) (2.886, 3.2979) (2.8647, 3.279) (2.845, 3.2588) (2.8265, 3.2376) (2.8097, 3.2149) (2.7945, 3.1911) (2.781, 3.1666) (2.7691, 3.1416) (2.759, 3.1163) (2.7511, 3.0905) (2.7445, 3.0645) (2.7399, 3.0382) (2.7373, 3.0114) (2.7369, 2.9934) (2.7367, 2.9844) knots 0 0 0 0 0.042841 0.085571 0.127719 0.170068 0.212787 0.255482 0.298877 0.342861 0.386528 0.429532 0.471886 0.513729 0.555082 0.596535 0.63812 0.679822 0.721331 0.761888 0.802199 0.841806 0.88106 0.920633 0.960101 1 1 1 1
  spline S242 degree 3 poles (2.7367, 2.9844) (2.7369, 2.9752) (2.7373, 2.9568) (2.7401, 2.9293) (2.7452, 2.9022) (2.752, 2.8755) (2.7606, 2.849) (2.7713, 2.8229) (2.7839, 2.7972) (2.7986, 2.7721) (2.8146, 2.7477) (2.8326, 2.7246) (2.8517, 2.7027) (2.8726, 2.6824) (2.8947, 2.6632) (2.9186, 2.6455) (2.9438, 2.6291) (2.9703, 2.6141) (2.998, 2.6007) (3.0264, 2.5888) (3.0555, 2.579) (3.0853, 2.5711) (3.1157, 2.5645) (3.1468, 2.5603) (3.1785, 2.5573) (3.1999, 2.557) (3.2106, 2.5569) knots 0 0 0 0 0.038994 0.077882 0.116652 0.155416 0.194618 0.234261 0.274547 0.315667 0.35702 0.398083 0.439098 0.479833 0.521274 0.562841 0.605292 0.648409 0.691727 0.735149 0.778369 0.821661 0.865524 0.909731 0.954523 1 1 1 1
  spline S243 degree 3 poles (3.2106, 2.5569) (3.2236, 2.5572) (3.249, 2.5577) (3.2865, 2.5619) (3.3224, 2.5683) (3.3568, 2.5778) (3.3896, 2.5899) (3.421, 2.6045) (3.4507, 2.6221) (3.4789, 2.642) (3.5048, 2.6641) (3.5282, 2.688) (3.5487, 2.7135) (3.5665, 2.7406) (3.5813, 2.7693) (3.5934, 2.7996) (3.6027, 2.8315) (3.6065, 2.8535) (3.6085, 2.8646) knots 0 0 0 0 0.07063 0.138694 0.204918 0.269441 0.332636 0.395302 0.457764 0.520657 0.582852 0.643315 0.70258 0.760908 0.81949 0.878269 0.938491 1 1 1 1
  line L288 (3.6085, 2.8646) -> (3.2751, 2.8646)
  line L289 (3.2751, 2.8646) -> (3.2751, 2.9672)
  line L290 (3.2751, 2.9672) -> (3.6982, 2.9672)
  spline S244 degree 3 poles (3.6982, 2.9672) (3.6977, 2.9481) (3.6968, 2.9106) (3.6901, 2.8561) (3.6793, 2.8046) (3.6645, 2.756) (3.6454, 2.7105) (3.6222, 2.668) (3.5944, 2.6287) (3.5631, 2.5924) (3.528, 2.56) (3.49, 2.5316) (3.4491, 2.5076) (3.4052, 2.4881) (3.3586, 2.4729) (3.3092, 2.4621) (3.2569, 2.4556) (3.2211, 2.4548) (3.2028, 2.4544) knots 0 0 0 0 0.071272 0.139493 0.204635 0.267406 0.328446 0.388397 0.447734 0.507392 0.566768 0.625478 0.684067 0.743248 0.804033 0.866499 0.931723 1 1 1 1
  spline S245 degree 3 poles (3.2028, 2.4544) (3.1915, 2.4545) (3.1693, 2.4548) (3.1364, 2.4571) (3.1044, 2.4606) (3.0733, 2.4659) (3.0431, 2.4724) (3.0137, 2.4807) (2.9853, 2.4903) (2.9576, 2.5013) (2.9309, 2.514) (2.9052, 2.5281) (2.8803, 2.5435) (2.8563, 2.5605) (2.8331, 2.579) (2.8109, 2.599) (2.7896, 2.6205) (2.7763, 2.6358) (2.7695, 2.6435) knots 0 0 0 0 0.069237 0.136557 0.202094 0.266464 0.329769 0.391879 0.453271 0.514115 0.57439 0.634142 0.693923 0.754152 0.81447 0.875661 0.937348 1 1 1 1
  spline S246 degree 3 poles (2.7695, 2.6435) (2.7598, 2.6557) (2.7404, 2.6798) (2.7154, 2.7186) (2.6942, 2.7587) (2.6769, 2.8003) (2.6635, 2.8433) (2.6538, 2.8878) (2.6482, 2.9336) (2.6473, 2.9647) (2.6469, 2.9804) knots 0 0 0 0 0.127896 0.253668 0.376738 0.499344 0.621999 0.745699 0.871345 1 1 1 1
  spline S247 degree 3 poles (7.9546, 5.7404) (7.9544, 5.7472) (7.9541, 5.7606) (7.9509, 5.7803) (7.9461, 5.7994) (7.9393, 5.8177) (7.9303, 5.8353) (7.9193, 5.852) (7.9066, 5.8682) (7.8919, 5.8834) (7.8758, 5.8973) (7.8588, 5.9097) (7.8408, 5.92) (7.8218, 5.9284) (7.8021, 5.935) (7.7814, 5.9396) (7.7599, 5.9425) (7.7452, 5.9429) (7.7377, 5.9431) knots 0 0 0 0 0.061965 0.122122 0.180988 0.239933 0.299906 0.359989 0.421776 0.486576 0.551535 0.615018 0.677259 0.73973 0.80305 0.866495 0.931973 1 1 1 1
  spline S248 degree 3 poles (7.7377, 5.9431) (7.7298, 5.9429) (7.7145, 5.9425) (7.6919, 5.9397) (7.6704, 5.9348) (7.6499, 5.9282) (7.6303, 5.9198) (7.6118, 5.9093) (7.5943, 5.8968) (7.578, 5.8826) (7.5629, 5.8668) (7.5496, 5.8492) (7.538, 5.8301) (7.5279, 5.8096) (7.5197, 5.7874) (7.5134, 5.7637) (7.5084, 5.7386) (7.5067, 5.7212) (7.5059, 5.7123) knots 0 0 0 0 0.064439 0.126547 0.186887 0.245878 0.304041 0.362191 0.420976 0.48066 0.5406 0.600689 0.661936 0.724443 0.789038 0.856314 0.926352 1 1 1 1
  line L291 (7.5059, 5.7123) -> (7.4162, 5.7123)
  spline S249 degree 3 poles (7.4162, 5.7123) (7.4167, 5.7242) (7.4179, 5.7476) (7.4233, 5.7817) (7.431, 5.8143) (7.4418, 5.8451) (7.4554, 5.8744) (7.4716, 5.9021) (7.4908, 5.9281) (7.5125, 5.9522) (7.5362, 5.9742) (7.5617, 5.9933) (7.5885, 6.0094) (7.6165, 6.0228) (7.6461, 6.0329) (7.6769, 6.0404) (7.7092, 6.0449) (7.7311, 6.0454) (7.7423, 6.0456) knots 0 0 0 0 0.068791 0.135103 0.198979 0.261904 0.323495 0.385195 0.446969 0.509765 0.572251 0.633405 0.693251 0.752583 0.812579 0.873275 0.93555 1 1 1 1
  spline S250 degree 3 poles (7.7423, 6.0456) (7.7532, 6.0454) (7.7748, 6.0449) (7.8062, 6.0405) (7.8362, 6.0338) (7.8645, 6.0242) (7.8911, 6.0114) (7.9161, 5.9961) (7.9398, 5.9783) (7.9611, 5.9574) (7.9807, 5.935) (7.9975, 5.9112) (8.012, 5.8865) (8.0241, 5.8609) (8.0329, 5.8341) (8.0397, 5.8065) (8.0435, 5.7777) (8.0441, 5.7583) (8.0444, 5.7484) knots 0 0 0 0 0.069475 0.136517 0.200789 0.26383 0.325735 0.387291 0.449509 0.512968 0.576275 0.63758 0.697903 0.757172 0.816599 0.876653 0.93729 1 1 1 1
  spline S251 degree 3 poles (8.0444, 5.7484) (8.0439, 5.7344) (8.0429, 5.7068) (8.0347, 5.6663) (8.0219, 5.6269) (8.0065, 5.5953) (7.9909, 5.5698) (7.9769, 5.5488) (7.9605, 5.5262) (7.9414, 5.5021) (7.9201, 5.4762) (7.8964, 5.4486) (7.8701, 5.4197) (7.8516, 5.3999) (7.842, 5.3896) knots 0 0 0 0 0.098702 0.195672 0.292422 0.391343 0.444462 0.504229 0.570352 0.642546 0.722288 0.807921 0.90047 1 1 1 1
  line L292 (7.842, 5.3896) -> (7.5918, 5.1226)
  line L293 (7.5918, 5.1226) -> (8.0572, 5.1226)
  line L294 (8.0572, 5.1226) -> (8.0572, 5.02)
  line L295 (8.0572, 5.02) -> (7.3777, 5.02)
  line L296 (7.3777, 5.02) -> (7.7655, 5.4339)
  spline S252 degree 3 poles (7.7655, 5.4339) (7.775, 5.4437) (7.7931, 5.4627) (7.8187, 5.4903) (7.8418, 5.5159) (7.8624, 5.5395) (7.88, 5.5614) (7.8957, 5.5809) (7.9083, 5.5988) (7.9219, 5.6196) (7.9351, 5.645) (7.9464, 5.676) (7.9534, 5.7079) (7.9542, 5.7295) (7.9546, 5.7404) knots 0 0 0 0 0.110803 0.212829 0.306101 0.390647 0.466924 0.534481 0.593587 0.644557 0.7362 0.825024 0.911986 1 1 1 1
  spline S253 degree 3 poles (7.2879, 5.5196) (7.2878, 5.5043) (7.2874, 5.4745) (7.2855, 5.4309) (7.2818, 5.3898) (7.2772, 5.351) (7.2708, 5.3147) (7.2629, 5.2808) (7.2541, 5.2491) (7.2433, 5.2198) (7.2315, 5.1927) (7.2186, 5.1674) (7.2048, 5.1436) (7.1898, 5.1216) (7.1738, 5.1012) (7.1564, 5.0828) (7.1382, 5.0659) (7.119, 5.0509) (7.0989, 5.0377) (7.0783, 5.0259) (7.0569, 5.0164) (7.0352, 5.0083) (7.0129, 5.002) (6.99, 4.9977) (6.9666, 4.9947) (6.9508, 4.9945) (6.9428, 4.9944) knots 0 0 0 0 0.065063 0.126773 0.185516 0.240765 0.29298 0.34225 0.388919 0.432776 0.474628 0.514775 0.553606 0.591426 0.628028 0.663804 0.698984 0.733591 0.767628 0.801208 0.834264 0.866981 0.89972 0.932702 0.966176 1 1 1 1
  spline S254 degree 3 poles (6.9428, 4.9944) (6.9349, 4.9945) (6.9194, 4.9948) (6.8963, 4.9975) (6.8739, 5.0018) (6.8521, 5.008) (6.8308, 5.0155) (6.8102, 5.0252) (6.7901, 5.0364) (6.7706, 5.0492) (6.752, 5.0639) (6.7343, 5.0801) (6.7178, 5.0983) (6.7025, 5.1182) (6.6879, 5.1395) (6.6745, 5.1626) (6.6622, 5.1874) (6.6508, 5.2141) (6.6408, 5.243) (6.6319, 5.2745) (6.6249, 5.3088) (6.6189, 5.3457) (6.6141, 5.3853) (6.6108, 5.4277) (6.6087, 5.4728) (6.6086, 5.5037) (6.6085, 5.5196) knots 0 0 0 0 0.033787 0.066622 0.099285 0.131361 0.163585 0.196104 0.228902 0.262158 0.295991 0.330218 0.36506 0.400951 0.43762 0.475708 0.515381 0.556414 0.599765 0.646424 0.696431 0.749782 0.806573 0.867436 0.931887 1 1 1 1
  spline S255 degree 3 poles (6.6085, 5.5196) (6.6086, 5.5356) (6.6087, 5.5668) (6.6108, 5.6121) (6.6141, 5.6547) (6.6187, 5.6944) (6.6243, 5.7314) (6.6318, 5.7655) (6.6404, 5.7968) (6.6502, 5.8255) (6.6614, 5.852) (6.6735, 5.8766) (6.6871, 5.8995) (6.7014, 5.921) (6.7169, 5.9407) (6.7333, 5.9589) (6.7511, 5.9751) (6.7698, 5.99) (6.7895, 6.0029) (6.8097, 6.0144) (6.8305, 6.0241) (6.8519, 6.0318) (6.8739, 6.0382) (6.8963, 6.0425) (6.9194, 6.0452) (6.9349, 6.0455) (6.9428, 6.0456) knots 0 0 0 0 0.068595 0.133246 0.194313 0.251279 0.304513 0.354235 0.400481 0.443411 0.484015 0.523252 0.561042 0.5979 0.633518 0.668314 0.702496 0.736685 0.770293 0.803437 0.835913 0.86846 0.900847 0.933467 0.966258 1 1 1 1
  spline S256 degree 3 poles (6.9428, 6.0456) (6.9507, 6.0455) (6.9666, 6.0452) (6.9899, 6.0426) (7.0128, 6.0381) (7.035, 6.0319) (7.0567, 6.0241) (7.0779, 6.0144) (7.0985, 6.003) (7.1183, 5.9897) (7.1375, 5.9749) (7.1556, 5.9581) (7.1727, 5.9395) (7.1889, 5.9194) (7.2038, 5.8973) (7.2179, 5.8737) (7.2306, 5.848) (7.2428, 5.8208) (7.2534, 5.7913) (7.2629, 5.7597) (7.2705, 5.7255) (7.2769, 5.689) (7.2819, 5.65) (7.2855, 5.6087) (7.2874, 5.5649) (7.2878, 5.535) (7.2879, 5.5196) knots 0 0 0 0 0.033788 0.067194 0.099862 0.132567 0.165151 0.197913 0.231319 0.265083 0.299255 0.334399 0.369943 0.406284 0.444064 0.482998 0.523354 0.565537 0.609613 0.656391 0.705885 0.758325 0.813832 0.872795 0.934722 1 1 1 1
  spline S257 degree 3 poles (3.5379, 5.0072) (3.5324, 5.0075) (3.5215, 5.0081) (3.5058, 5.013) (3.4914, 5.0206) (3.4786, 5.0313) (3.4682, 5.0441) (3.4603, 5.0585) (3.4556, 5.0741) (3.4549, 5.085) (3.4546, 5.0905) knots 0 0 0 0 0.127757 0.249414 0.372796 0.500111 0.62861 0.750643 0.873768 1 1 1 1
  spline S258 degree 3 poles (3.4546, 5.0905) (3.4549, 5.0962) (3.4555, 5.1072) (3.4603, 5.1229) (3.4681, 5.1373) (3.4787, 5.15) (3.4914, 5.1606) (3.5058, 5.1683) (3.5215, 5.1729) (3.5324, 5.1735) (3.5379, 5.1738) knots 0 0 0 0 0.129097 0.252046 0.373905 0.501038 0.628171 0.751376 0.872426 1 1 1 1
  spline S259 degree 3 poles (3.5379, 5.1738) (3.5435, 5.1735) (3.5544, 5.1729) (3.5702, 5.1684) (3.5845, 5.1605) (3.5972, 5.15) (3.6077, 5.1372) (3.6159, 5.123) (3.6203, 5.1071) (3.621, 5.0961) (3.6213, 5.0905) knots 0 0 0 0 0.127519 0.249986 0.371792 0.49887 0.625948 0.748492 0.870959 1 1 1 1
  spline S260 degree 3 poles (3.6213, 5.0905) (3.6209, 5.085) (3.6203, 5.0742) (3.6159, 5.0584) (3.6076, 5.0442) (3.5973, 5.0313) (3.5845, 5.0207) (3.5702, 5.0129) (3.5545, 5.0081) (3.5435, 5.0075) (3.5379, 5.0072) knots 0 0 0 0 0.126178 0.248821 0.37154 0.499984 0.627244 0.749226 0.872298 1 1 1 1
  line L297 (2.7238, 5.52) -> (2.8264, 6.02)
  line L298 (2.8264, 6.02) -> (3.2367, 6.02)
  line L299 (3.2367, 6.02) -> (3.2367, 5.9174)
  line L300 (3.2367, 5.9174) -> (2.8965, 5.9174)
  line L301 (2.8965, 5.9174) -> (2.8426, 5.6544)
  spline S261 degree 3 poles (2.8426, 5.6544) (2.8532, 5.6573) (2.8737, 5.663) (2.904, 5.6693) (2.9327, 5.6731) (2.9514, 5.6736) (2.9604, 5.6738) knots 0 0 0 0 0.275068 0.532901 0.773973 1 1 1 1
  spline S262 degree 3 poles (2.9604, 5.6738) (2.9716, 5.6736) (2.9935, 5.6731) (3.0257, 5.6686) (3.0563, 5.6614) (3.0855, 5.6513) (3.1132, 5.6385) (3.1391, 5.6225) (3.1637, 5.6038) (3.1866, 5.5822) (3.2073, 5.5585) (3.2255, 5.5331) (3.241, 5.5061) (3.2534, 5.4773) (3.2634, 5.447) (3.27, 5.4149) (3.2744, 5.3814) (3.2749, 5.3584) (3.2751, 5.3467) knots 0 0 0 0 0.065808 0.129394 0.190894 0.251281 0.310815 0.370371 0.430768 0.492881 0.555104 0.616067 0.677256 0.73826 0.800762 0.864778 0.931045 1 1 1 1
  spline S263 degree 3 poles (3.2751, 5.3467) (3.2749, 5.3386) (3.2746, 5.3224) (3.2726, 5.2983) (3.2689, 5.2748) (3.264, 5.2518) (3.2575, 5.2293) (3.2497, 5.2073) (3.2402, 5.1859) (3.2297, 5.165) (3.218, 5.1449) (3.2049, 5.1262) (3.1911, 5.1084) (3.1762, 5.0919) (3.1601, 5.0767) (3.1431, 5.0627) (3.1252, 5.0497) (3.1061, 5.0382) (3.0864, 5.0277) (3.0656, 5.019) (3.0443, 5.0113) (3.0222, 5.0051) (2.9994, 5.0003) (2.9757, 4.997) (2.9513, 4.9946) (2.9347, 4.9944) (2.9264, 4.9944) knots 0 0 0 0 0.044014 0.087434 0.130118 0.172554 0.214555 0.256298 0.298438 0.340849 0.382715 0.423924 0.464246 0.504074 0.543862 0.583567 0.623094 0.663229 0.703551 0.743938 0.784541 0.82575 0.867757 0.910745 0.954914 1 1 1 1
  spline S264 degree 3 poles (2.9264, 4.9944) (2.9164, 4.9946) (2.8968, 4.9949) (2.8681, 4.999) (2.8405, 5.0048) (2.8141, 5.0136) (2.7889, 5.0245) (2.765, 5.0384) (2.742, 5.0541) (2.7207, 5.0727) (2.701, 5.0929) (2.6833, 5.1149) (2.6675, 5.1383) (2.654, 5.1631) (2.6424, 5.1893) (2.6333, 5.2171) (2.626, 5.2462) (2.6229, 5.2662) (2.6213, 5.2764) knots 0 0 0 0 0.065421 0.128708 0.190236 0.250724 0.310637 0.370766 0.431615 0.493523 0.555883 0.617342 0.678668 0.740711 0.802985 0.866803 0.932347 1 1 1 1
  line L302 (2.6213, 5.2764) -> (2.711, 5.2764)
  spline S265 degree 3 poles (2.711, 5.2764) (2.7132, 5.2669) (2.7175, 5.2485) (2.7268, 5.2228) (2.7382, 5.1998) (2.7517, 5.1794) (2.7679, 5.1616) (2.7863, 5.1457) (2.807, 5.1313) (2.83, 5.1194) (2.8542, 5.1092) (2.8796, 5.1024) (2.9054, 5.0976) (2.9228, 5.0972) (2.9316, 5.0969) knots 0 0 0 0 0.094687 0.181994 0.264377 0.34218 0.418618 0.496509 0.577369 0.661511 0.746733 0.831258 0.915206 1 1 1 1
  spline S266 degree 3 poles (2.9316, 5.0969) (2.9401, 5.0972) (2.957, 5.0976) (2.9818, 5.1012) (3.0057, 5.1066) (3.0286, 5.1148) (3.0508, 5.1248) (3.0717, 5.1376) (3.0919, 5.1523) (3.1109, 5.1691) (3.1283, 5.1877) (3.1436, 5.2075) (3.1564, 5.2287) (3.1672, 5.2508) (3.1754, 5.2742) (3.1812, 5.2986) (3.1847, 5.3242) (3.1851, 5.3416) (3.1854, 5.3505) knots 0 0 0 0 0.064207 0.126425 0.18768 0.248216 0.308305 0.369661 0.431699 0.495947 0.559758 0.622295 0.683911 0.745092 0.80674 0.869087 0.93329 1 1 1 1
  spline S267 degree 3 poles (3.1854, 5.3505) (3.1852, 5.3586) (3.1848, 5.3743) (3.1818, 5.3972) (3.1766, 5.419) (3.1693, 5.4396) (3.1601, 5.4591) (3.1488, 5.4775) (3.1353, 5.4945) (3.1198, 5.5103) (3.1029, 5.5248) (3.0842, 5.5372) (3.0641, 5.5476) (3.0429, 5.5566) (3.0201, 5.563) (2.9961, 5.5679) (2.9706, 5.5707) (2.9532, 5.5711) (2.9442, 5.5713) knots 0 0 0 0 0.065351 0.127916 0.18836 0.247216 0.30563 0.36377 0.422661 0.482687 0.5433 0.604118 0.664965 0.727413 0.791468 0.858055 0.927037 1 1 1 1
  spline S268 degree 3 poles (2.9442, 5.5713) (2.9364, 5.5711) (2.9204, 5.5708) (2.8959, 5.5683) (2.8701, 5.5642) (2.8431, 5.5586) (2.815, 5.5513) (2.7856, 5.5425) (2.755, 5.532) (2.7344, 5.5241) (2.7238, 5.52) knots 0 0 0 0 0.102203 0.211023 0.3251 0.446502 0.573788 0.708901 0.850358 1 1 1 1
  line L303 (-4.4546, -12.76) -> (-4.5444, -12.76)
  line L304 (-4.5444, -12.76) -> (-4.5444, -11.76)
  line L305 (-4.5444, -11.76) -> (-4.3442, -11.76)
  spline S269 degree 3 poles (-4.3442, -11.76) (-4.3309, -11.76) (-4.3052, -11.7601) (-4.2685, -11.7606) (-4.2351, -11.762) (-4.2051, -11.7631) (-4.1785, -11.7653) (-4.1552, -11.7673) (-4.1352, -11.77) (-4.1231, -11.7725) (-4.1177, -11.7736) knots 0 0 0 0 0.176258 0.338434 0.484822 0.617158 0.734698 0.837385 0.926372 1 1 1 1
  spline S270 degree 3 poles (-4.1177, -11.7736) (-4.1104, -11.7754) (-4.0959, -11.779) (-4.075, -11.7866) (-4.0552, -11.7953) (-4.0364, -11.8056) (-4.0187, -11.8175) (-4.0021, -11.8307) (-3.9863, -11.8453) (-3.9721, -11.8616) (-3.9587, -11.8787) (-3.9474, -11.8972) (-3.9376, -11.9166) (-3.9299, -11.9369) (-3.9236, -11.9581) (-3.9192, -11.9804) (-3.9166, -12.0036) (-3.9163, -12.0194) (-3.9162, -12.0274) knots 0 0 0 0 0.064217 0.127064 0.188745 0.249132 0.309453 0.369827 0.43065 0.492352 0.554072 0.61569 0.676798 0.738439 0.801317 0.865185 0.931641 1 1 1 1
  spline S271 degree 3 poles (-3.9162, -12.0274) (-3.9166, -12.0408) (-3.9174, -12.0668) (-3.925, -12.1045) (-3.9375, -12.1397) (-3.9548, -12.1723) (-3.9767, -12.2017) (-4.0031, -12.2275) (-4.0339, -12.2491) (-4.0626, -12.2641) (-4.088, -12.2737) (-4.1088, -12.2805) (-4.1316, -12.2857) (-4.156, -12.2904) (-4.1822, -12.2939) (-4.2102, -12.2965) (-4.2399, -12.2981) (-4.2602, -12.2983) (-4.2707, -12.2985) knots 0 0 0 0 0.07878 0.153721 0.226714 0.299191 0.37119 0.443006 0.516689 0.593217 0.633873 0.676989 0.7229 0.771959 0.824211 0.879379 0.937948 1 1 1 1
  line L306 (-4.2707, -12.2985) -> (-3.9033, -12.76)
  line L307 (-3.9033, -12.76) -> (-4.0143, -12.76)
  line L308 (-4.0143, -12.76) -> (-4.3817, -12.2985)
  line L309 (-4.3817, -12.2985) -> (-4.4546, -12.2985)
  line L310 (-4.4546, -12.2985) -> (-4.4546, -12.76)
  spline S272 degree 3 poles (-4.429, -9.975) (-4.4292, -9.984) (-4.4295, -10.0017) (-4.4338, -10.0278) (-4.4401, -10.0531) (-4.4495, -10.0774) (-4.461, -10.101) (-4.4757, -10.1234) (-4.4926, -10.1451) (-4.512, -10.1654) (-4.5333, -10.1841) (-4.5558, -10.2007) (-4.5795, -10.2146) (-4.6044, -10.2259) (-4.6303, -10.2347) (-4.6574, -10.2411) (-4.6857, -10.245) (-4.7049, -10.2454) (-4.7146, -10.2456) knots 0 0 0 0 0.061484 0.121775 0.18092 0.240256 0.300114 0.361146 0.423501 0.488669 0.553954 0.617581 0.680238 0.742187 0.804663 0.868259 0.93302 1 1 1 1
  spline S273 degree 3 poles (-4.7146, -10.2456) (-4.7222, -10.2455) (-4.7372, -10.2452) (-4.7594, -10.2426) (-4.7812, -10.239) (-4.8022, -10.2332) (-4.8228, -10.2263) (-4.8428, -10.2176) (-4.8623, -10.2073) (-4.8814, -10.1955) (-4.9, -10.1818) (-4.918, -10.1658) (-4.9359, -10.148) (-4.9533, -10.1279) (-4.9704, -10.1058) (-4.9869, -10.0815) (-5.0032, -10.0552) (-5.0135, -10.0366) (-5.0187, -10.0271) knots 0 0 0 0 0.057208 0.113696 0.169178 0.224159 0.27872 0.333794 0.389241 0.445822 0.503704 0.564294 0.627975 0.695038 0.765373 0.839611 0.917538 1 1 1 1
  line L311 (-5.0187, -10.0271) -> (-4.9342, -9.9764)
  spline S274 degree 3 poles (-4.9342, -9.9764) (-4.9263, -9.9896) (-4.9113, -10.0148) (-4.8861, -10.0489) (-4.8601, -10.0778) (-4.8329, -10.1015) (-4.8049, -10.1201) (-4.7757, -10.1333) (-4.7455, -10.1416) (-4.7249, -10.1426) (-4.7146, -10.1431) knots 0 0 0 0 0.159004 0.304646 0.438547 0.562322 0.677433 0.786897 0.893611 1 1 1 1
  spline S275 degree 3 poles (-4.7146, -10.1431) (-4.7059, -10.1428) (-4.6885, -10.1423) (-4.6629, -10.1377) (-4.638, -10.1306) (-4.6144, -10.1203) (-4.5924, -10.1079) (-4.5731, -10.093) (-4.5564, -10.0762) (-4.5427, -10.0576) (-4.5323, -10.0375) (-4.5242, -10.0168) (-4.5197, -9.9954) (-4.5191, -9.9809) (-4.5187, -9.9736) knots 0 0 0 0 0.091264 0.18093 0.270088 0.360156 0.448343 0.532666 0.613834 0.693982 0.772716 0.849335 0.923967 1 1 1 1
  spline S276 degree 3 poles (-4.5187, -9.9736) (-4.5191, -9.9653) (-4.52, -9.9484) (-4.5272, -9.9234) (-4.5386, -9.8987) (-4.5491, -9.8834) (-4.5546, -9.8754) knots 0 0 0 0 0.234723 0.477158 0.728556 1 1 1 1
  spline S277 degree 3 poles (-4.5546, -9.8754) (-4.5591, -9.8697) (-4.5685, -9.8577) (-4.5846, -9.8398) (-4.6036, -9.8213) (-4.6247, -9.8016) (-4.6487, -9.7815) (-4.6749, -9.7601) (-4.704, -9.7382) (-4.7244, -9.7236) (-4.7349, -9.716) knots 0 0 0 0 0.090279 0.18953 0.299198 0.418926 0.548376 0.688136 0.839084 1 1 1 1
  spline S278 degree 3 poles (-4.7349, -9.716) (-4.7454, -9.7085) (-4.7655, -9.6942) (-4.7936, -9.6729) (-4.8188, -9.6535) (-4.8409, -9.6357) (-4.8598, -9.6195) (-4.8759, -9.6051) (-4.8885, -9.5922) (-4.8956, -9.5838) (-4.8987, -9.58) knots 0 0 0 0 0.181535 0.347082 0.495568 0.628357 0.74552 0.845831 0.930782 1 1 1 1
  spline S279 degree 3 poles (-4.8987, -9.58) (-4.9031, -9.5741) (-4.9118, -9.5625) (-4.9233, -9.5444) (-4.9331, -9.5259) (-4.9407, -9.5069) (-4.9472, -9.4877) (-4.9515, -9.468) (-4.9542, -9.448) (-4.9545, -9.4345) (-4.9546, -9.4277) knots 0 0 0 0 0.133507 0.262559 0.388264 0.512667 0.633722 0.755394 0.877553 1 1 1 1
  spline S280 degree 3 poles (-4.9546, -9.4277) (-4.9542, -9.4172) (-4.9535, -9.3962) (-4.9473, -9.3656) (-4.9374, -9.3364) (-4.9236, -9.3089) (-4.9058, -9.2838) (-4.8852, -9.2608) (-4.8607, -9.2414) (-4.8338, -9.2245) (-4.8044, -9.2112) (-4.7735, -9.2012) (-4.7412, -9.1956) (-4.7193, -9.1948) (-4.7082, -9.1944) knots 0 0 0 0 0.083785 0.16578 0.24628 0.327461 0.408797 0.489715 0.571376 0.655523 0.741019 0.826547 0.911989 1 1 1 1
  spline S281 degree 3 poles (-4.7082, -9.1944) (-4.6964, -9.1948) (-4.673, -9.1956) (-4.6385, -9.2026) (-4.6053, -9.2142) (-4.5786, -9.2274) (-4.5577, -9.2406) (-4.5418, -9.2526) (-4.5257, -9.2664) (-4.5092, -9.2821) (-4.4926, -9.2998) (-4.4758, -9.3193) (-4.4585, -9.3406) (-4.4475, -9.3558) (-4.4418, -9.3636) knots 0 0 0 0 0.107233 0.213252 0.31883 0.426794 0.483646 0.543604 0.608308 0.677127 0.750686 0.828713 0.91219 1 1 1 1
  line L312 (-4.4418, -9.3636) -> (-4.5229, -9.4251)